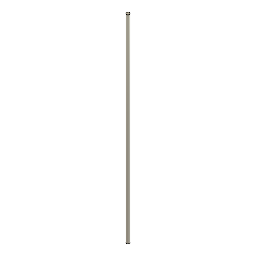
8mm Smooth Rod 481mm (Autodesk Fusion 360 design; units mm, degrees)
Autodesk Fusion 360 part; units mm, degrees
form "Form1" [no effect]
cylinder "CylinderPrimitive1" add diameter 8 height 300 placed x (1, 0, 0) y (0, 0, -1) z (0, 1, 0) at (0, 0, 0)
move_face "OffsetFaces1" offset 36 1 faces at (-1.2456, 300, -0.0132)
move_face "OffsetFaces2" offset 145 1 faces at (-1.2456, 0, -0.0132)
